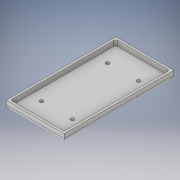
# Autodesk Inventor part: Motor_Node_top
Saved by Autodesk Inventor 2019 (Build 230136000, 136)
## iProperties
Created: 2019-12-12
Part Number: Motor_Node_top
Material: Generic
Document SubType Name: Modeling
Designer: Jorian Brusind
Density: 1 g/cm^3
Appearance: Default
Author: Jorian Brusind
Autodesk Inventor part; units mm, degrees
ref_plane "YZ Plane" through (0, 0, 0) normal (1, 0, 0) x (0, 1, 0)
ref_plane "XZ Plane" through (0, 0, 0) normal (0, 1, 0) x (-1, 0, 0)
ref_plane "XY Plane" through (0, 0, 0) normal (0, 0, 1) x (1, 0, 0)
sketch "Sketch1" plane through (0, 0, 0) normal (0, 1, 0) x (-1, 0, 0)
  line L0 (-28, 53) -> (28, 53)
  line L1 (28, 53) -> (28, -53)
  line L2 (28, -53) -> (-28, -53)
  line L3 (-28, -53) -> (-28, 53)
  line L4 (-28, 53) -> (28, -53) construction
  line L5 (28, 53) -> (-28, -53) construction
  point P0 (0, 0)
  dimension "d0" = 56
  dimension "d1" = 106
  constraints: 12 end point, 2 midpoint, 2 parallel, 1 horizontal, 1 perpendicular
  measures "d0" distance of L1.end L2.end
  measures "d1" distance of L0.end L1.end
extrude "Extrusion1" add sketch "Sketch1" along normal blind 3
sketch "Sketch2" plane through (0, 3, 0) normal (0, 1, 0) x (1, 0, 0)
  line L0 (-28, 53) -> (-28, -53) projected
  line L1 (28, 53) -> (-28, 53)
  line L2 (-28, 53) -> (-28, -53)
  line L3 (-28, -53) -> (28, -53)
  line L4 (28, -53) -> (28, 53)
  line L5 (28, 53) -> (-28, -53) construction
  line L6 (-28, 53) -> (28, -53) construction
  line L7 (26, 51) -> (-26, 51)
  line L8 (-26, 51) -> (-26, -51)
  line L9 (-26, -51) -> (26, -51)
  line L10 (26, -51) -> (26, 51)
  line L11 (26, 51) -> (-26, -51) construction
  line L12 (-26, 51) -> (26, -51) construction
  point P0 (0, 0)
  dimension "d4" = 52
  dimension "d5" = 102
  constraints: 24 end point, 4 midpoint, 4 parallel, 2 horizontal, 2 perpendicular
  measures "d4" distance of L9.end L8.end
  measures "d5" distance of L8.end L7.end
extrude "Extrusion2" add sketch "Sketch2" along normal blind 5
sketch "Sketch3" plane through (0, 3, 0) normal (0, 1, 0) x (1, 0, 0)
  circle A0 centre (15, 32) radius 1.75
  line L0 (-26, 51) -> (26, 51) projected
  line L1 (26, 51) -> (26, -51) projected
  circle A1 centre (15, -32) radius 1.75
  circle A2 centre (-15, 32) radius 1.75
  circle A3 centre (-15, -32) radius 1.75
  point P0 (0, 0)
  dimension "d8" = 3.5
  dimension "d9" = 19
  dimension "d10" = 11
  dimension "d13" = 64
  dimension "d16" = 30
  constraints: 4 centre point, 1 horizontal, 1 vertical, 6 other
  measures "d8" diameter of A0
  measures "d9" distance from line of L0 A0.centre
  measures "d10" distance from line of L1 A0.centre
  measures "d13" distance of A0.centre A1.centre
  measures "d16" distance of A0.centre A2.centre
extrude "Extrusion3" cut sketch "Sketch3" against normal blind 5
fillet "Fillet1" radius 4 4 edges at (28, 0, 0) (-28, 0, 0) (0, 0, 53) (0, 0, -53)
fillet "Fillet2" radius 2 4 edges at (-26, 5.5, -51) (26, 5.5, -51) (26, 5.5, 51) (-26, 5.5, 51)
body "Solid1"
